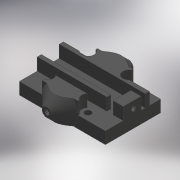
# Autodesk Inventor part: Platine
Saved by Autodesk Inventor 2017 (Build 210142000, 142)
## iProperties
Part Number: Platine
Material: Aluminium
Document SubType Name: Modeling
Designer: FABLAB Frenchmakers
Density: 2.7 g/cm^3
Appearance: Par défaut(1)
Mass: 25.7328 g
Surface Area: 52.6897 cm^2
Volume: 9.53068 cm^3
Project: 1420 Vauban 3D XL
Catalog Web Link: http://frenchmakers.com/
Stock Number: 1420-12-04
Author: FABLAB Frenchmakers
Autodesk Inventor part; units mm, degrees
ref_plane "YZ Plane" through (0, 0, 0) normal (1, 0, 0) x (0, 1, 0)
ref_plane "XZ Plane" through (0, 0, 0) normal (0, 1, 0) x (-1, 0, 0)
sketch "Esquisse1" plane through (0, 0, 0) normal (0, 0, 1) x (1, 0, 0)
  line L0 (-21, -13.5) -> (21, -13.5)
  line L1 (21, -13.5) -> (21, 13.5)
  line L2 (21, 13.5) -> (-21, 13.5)
  line L3 (-21, 13.5) -> (-21, -13.5)
  line L4 (-21, -13.5) -> (21, 13.5) construction
  line L5 (21, -13.5) -> (-21, 13.5) construction
  point P0 (0, 0)
  dimension "d0" = 42
  dimension "d1" = 27
  constraints: 12 end point, 2 midpoint, 2 parallel, 1 horizontal, 1 perpendicular
  measures "d0" distance of L2.end L1.end
  measures "d1" distance of L1.end L0.end
extrude "Extrusion1" add sketch "Esquisse1" along normal mid plane 5.75
sketch "Esquisse2" plane through (0, 0, 2.875) normal (0, 0, 1) x (1, 0, 0)
  line L0 (16, -4.75) -> (21, -4.75)
  line L1 (21, -4.75) -> (21, 4)
  line L2 (21, 4) -> (16, 4)
  line L3 (16, 4) -> (16, -4.75)
  line L4 (-21, 6) -> (21, 6)
  line L5 (21, 6) -> (21, 8)
  line L6 (21, 8) -> (-21, 8)
  line L7 (-21, 8) -> (-21, 6)
  line L8 (-21, -4.75) -> (13, -4.75)
  line L9 (13, -4.75) -> (13, -2.75)
  line L10 (13, -2.75) -> (-21, -2.75)
  line L11 (-21, -2.75) -> (-21, -4.75)
  line L12 (-21, -13.5) -> (21, -13.5) construction
  line L13 (21, -13.5) -> (21, 13.5) construction
  line L14 (21, 13.5) -> (-21, 13.5) construction
  line L15 (-21, 13.5) -> (-21, -13.5) construction
  point P0 (0, 0)
  dimension "d4" = 2
  dimension "d5" = 2
  dimension "d6" = 5
  dimension "d7" = 8.75
  dimension "d8" = 2
  dimension "d9" = 5.5
  dimension "d10" = 34
  constraints: 24 end point, 6 parallel, 5 collinear, 3 horizontal, 3 perpendicular
  measures "d4" distance of L8.end L9.end
  measures "d5" distance between parallel lines of L6 L4
  measures "d6" distance of L0.start L0.end
  measures "d7" distance of L2.end L0.start
  measures "d8" distance between parallel lines of L4 L2
  measures "d9" distance between parallel lines of L14 L6
  measures "d10" distance of L8.start L8.end
extrude "Extrusion2" add sketch "Esquisse2" along normal blind 6
sketch "Esquisse3" plane through (0, 0, 2.875) normal (0, 0, 1) x (1, 0, 0)
  line L0 (-9.85, 8) -> (7.55, 8)
  line L1 (7.55, 8) -> (7.55, 13.5)
  line L2 (7.55, 13.5) -> (-9.85, 13.5)
  line L3 (-9.85, 13.5) -> (-9.85, 8)
  line L4 (-21, 6) -> (21, 6) construction
  line L5 (21, 6) -> (21, 8) construction
  line L6 (21, 8) -> (-21, 8) construction
  line L7 (-21, 8) -> (-21, 6) construction
  line L8 (-21, 8) -> (21, 8) construction
  line L9 (21, 8) -> (21, 13.5) construction
  line L10 (21, 13.5) -> (-21, 13.5) construction
  line L11 (-21, 13.5) -> (-21, 8) construction
  line L12 (21, 8) -> (-21, 8) construction
  line L13 (-21, -13.5) -> (21, -13.5) projected
  line L14 (-9.85, -13.5) -> (7.55, -13.5)
  line L15 (7.55, -13.5) -> (7.55, -8.05)
  line L16 (7.55, -8.05) -> (-9.85, -8.05)
  line L17 (-9.85, -8.05) -> (-9.85, -13.5)
  line L18 (-21, -4.75) -> (13, -4.75) projected
  point P0 (0, 0)
  dimension "d13" = 17.4
  dimension "d14" = 11.15
  dimension "d17" = 3.3
  constraints: 16 end point, 4 collinear, 4 parallel, 2 horizontal, 2 perpendicular, 1 point on line
  measures "d13" distance between parallel lines of L3 L1
  measures "d14" distance between parallel lines of L11 L3
  measures "d17" distance between parallel lines of L18 L16
extrude "Extrusion3" add sketch "Esquisse3" along normal up to surface (6 mm away)
ref_plane "Plan de construction1" through (-9.85, -13.5, 3) normal (0, 0, 1) x (1, 0, 0)
sketch "Esquisse5" plane through (-9.85, -13.5, 3) normal (0, 0, 1) x (1, 0, 0)
  line L0 (8.7, 27) -> (8.7, 37.7161)
  line L1 (0, 27) -> (17.4, 27) projected
  line L2 (0, 27) -> (6.45, 33.5)
  line L3 (6.45, 33.5) -> (8.7, 33.5)
  line L4 (0, 27) -> (8.7, 27)
  line L5 (-11.15, 27) -> (30.85, 27) projected
  point P0 (9.85, 13.5)
  dimension "d18" = 4.5
  dimension "d19" = 6.5
  constraints: 8 end point, 1 collinear, 1 midpoint, 1 perpendicular, 1 point on line, 1 vertical
  measures "d18" diameter of L2.end L0
  measures "d19" distance between parallel lines of L3 L1
revolve "Révolution1" add sketch "Esquisse5" angle 360 about axis through (-1.15, 13.5, 3) along (0, 1, 0)
sketch "Esquisse7" plane through (-1.15, 20, 3) normal (0, 1, 0) x (1, 0, 0)
  circle A0 centre (0, 0) radius 2.25 construction
  point P0 (1.15, 3)
  constraints: 1 coincident
hole "Perçage1" at (-1.15, 20, 3) direction (0, -1, 0) diameter 2.459 depth 11 tip angle 118 thread size "M3x0.5" class "6H" standard "ISO Metric profile"
mirror "Symétrie2" about plane through (0, 0, 0) normal (0, 1, 0) of "Révolution1", "Perçage1"
sketch "Esquisse6" plane through (0, 0, 0) normal (0, 1, 0) x (-1, 0, 0)
  line L0 (7.5667, 8.875) -> (-5.2667, 8.875) projected
  arc A0 (7.5667, 8.875) -> (-5.2667, 8.875) centre (1.15, 3) ccw projected
  line L1 (7.5667, -2.875) -> (-5.2667, -2.875) projected
  arc A1 (-5.2667, -2.875) -> (7.5667, -2.875) centre (1.15, 3) ccw projected
  point P0 (0, 0)
extrude "Extrusion4" cut sketch "Esquisse6" along normal through all both and the other way through all
sketch "Esquisse8" plane through (-21, -13.5, -2.875) normal (-1, 0, 0) x (0, 0, 1)
  point P0 (2.875, 13.5)
  point P1 (2.875, 13.5)
  constraints: 1 coincident
hole "Perçage2" at (-21, 0, 0) direction (1, 0, 0) diameter 2.459 depth 6 tip angle 118 thread size "M3x0.5" class "6H" standard "ISO Metric profile"
sketch "Esquisse9" plane through (21, -13.5, -2.875) normal (1, 0, 0) x (0, 0, -1)
  line L0 (-11.75, 8.75) -> (-11.75, 17.5) projected
  line L1 (-5.75, 17.5) -> (-11.75, 17.5) projected
  point P0 (-2.875, 13.5)
  point P1 (-8.35, 13.95)
  dimension "d37" = 3.4
  dimension "d38" = 3.55
  measures "d37" distance from line of L0 point (-8.35, 13.95)
  measures "d38" distance from line of L1 point (-8.35, 13.95)
hole "Perçage3" at (21, 0.45, 5.475) direction (-1, 0, 0) diameter 2.459 end through all thread size "M3x0.5" class "6H" standard "ISO Metric profile"
sketch "Esquisse10" plane through (0, 0, -2.875) normal (0, 0, -1) x (-1, 0, 0)
  line L0 (21, -13.5) -> (21, 13.5) projected
  point P0 (0, 0)
  point P1 (-9, -10)
  point P2 (-9, 10)
  point P3 (11, 10)
  point P4 (11, -10)
  dimension "d46" = 20
  dimension "d47" = 20
  dimension "d48" = 10
  dimension "d49" = 10
  constraints: 2 horizontal alignment, 2 vertical alignment
  measures "d46" distance of point (11, 10) point (-9, 10)
  measures "d47" distance of point (11, -10) point (11, 10)
  measures "d48" vertical distance of point (0, 0) point (11, 10)
  measures "d49" distance from line of L0 point (11, 10)
hole "Perçage4" at (9, -10, -2.875) at (9, 10, -2.875) at (-11, 10, -2.875) at (-11, -10, -2.875) direction (0, 0, 1) diameter 3 end through all
sketch "Esquisse11" plane through (0, 0, -2.875) normal (0, 0, -1) x (-1, 0, 0)
  line L0 (21, -13.5) -> (21, 13.5) projected
  line L1 (21, 13.5) -> (7.5667, 13.5) projected
  point P0 (0, 0)
  point P1 (-5.5, 1.6)
  point P2 (12.75, 1.6)
  dimension "d57" = 18.25
  dimension "d58" = 8.25
  dimension "d59" = 11.9
  constraints: 1 horizontal alignment
  measures "d57" distance of point (12.75, 1.6) point (-5.5, 1.6)
  measures "d58" distance from line of L0 point (12.75, 1.6)
  measures "d59" distance from line of L1 point (12.75, 1.6)
hole "Perçage5" at (5.5, 1.6, -2.875) at (-12.75, 1.6, -2.875) direction (0, 0, 1) diameter 2.459 end through all thread size "M3x0.5" class "6H" standard "ISO Metric profile"
sketch "Esquisse12" plane through (-9.85, -8.05, 8.875) normal (0, 0, 1) x (1, 0, 0)
  arc A0 (17.4, -2.3341) -> (17.4, -1.5659) centre (18.85, -1.95) ccw construction
  arc A1 (0, -0.9869) -> (0, -2.9131) centre (-1.15, -1.95) ccw construction
  arc A2 (0, 19.0131) -> (0, 17.0869) centre (-1.15, 18.05) ccw construction
  arc A3 (17.4, 17.6659) -> (17.4, 18.4341) centre (18.85, 18.05) ccw construction
  circle A4 centre (18.85, -1.95) radius 3
  circle A5 centre (-1.15, -1.95) radius 1.5 projected
  circle A6 centre (-1.15, -1.95) radius 3
  circle A7 centre (-1.15, 18.05) radius 3
  circle A8 centre (18.85, 18.05) radius 1.5 projected
  circle A9 centre (18.85, 18.05) radius 3
  point P0 (9.85, 8.05)
  dimension "d67" = 6
  dimension "d68" = 6
  dimension "d69" = 6
  dimension "d70" = 6
  constraints: 4 centre point, 4 coincident
  measures "d67" diameter of A4
  measures "d68" diameter of A6
  measures "d69" diameter of A9
  measures "d70" diameter of A7
extrude "Extrusion5" cut sketch "Esquisse12" against normal up to surface (6 mm away)
equation "\"d48\" = 0.5 * d47"
equation "\"d68\" = d67"
equation "\"d69\" = d67"
equation "\"d70\" = d68"
